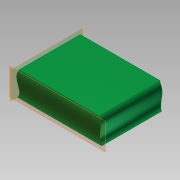
# Autodesk Inventor part: GP-WSM010 board
Saved by Autodesk Inventor 2011 (Build 150239000, 239)
## iProperties
Created: 2010-12-28
Part Number: GP-WSM010 board
Document SubType Name: Modeling
Designer: abbath
Density: 1 g/cm^3
Mass: 0.0283841 g
Surface Area: 0.648912 cm^2
Volume: 0.0283841 cm^3
Author: abbath
Autodesk Inventor part; units mm, degrees
ref_plane "YZ Plane" through (0, 0, 0) normal (1, 0, 0) x (0, 1, 0)
ref_plane "XZ Plane" through (0, 0, 0) normal (0, 1, 0) x (-1, 0, 0)
ref_plane "XY Plane" through (0, 0, 0) normal (0, 0, 1) x (1, 0, 0)
sketch "Эскиз1" plane through (0, 0, 0) normal (0, 0, 1) x (1, 0, 0)
  line L0 (-2.365, 1.705) -> (-2.365, -1.705) projected
  line L1 (-2.365, -1.705) -> (-1.665, -1.705) projected
  line L2 (2.365, 1.705) -> (1.665, 1.705) projected
  line L3 (2.365, -1.705) -> (2.365, 1.705) projected
  line L4 (-2.665, -2.005) -> (2.665, -2.005)
  line L5 (2.665, -2.005) -> (2.665, 2.005)
  line L6 (2.665, 2.005) -> (-2.665, 2.005)
  line L7 (-2.665, 2.005) -> (-2.665, -2.005)
  point P0 (0, 0)
  dimension "d0" = 0.3
  dimension "d1" = 0.3
  dimension "d2" = 0.3
  dimension "d3" = 0.3
  constraints: 8 end point, 2 parallel, 1 horizontal, 1 perpendicular
  measures "d0" distance between parallel lines of L0 L7
  measures "d1" distance between parallel lines of L4 L1
  measures "d2" distance between parallel lines of L6 L2
  measures "d3" distance between parallel lines of L5 L3
extrude "Выдавливание1" add sketch "Эскиз1" along normal blind 1.5
ref_plane "РабПлоскость1" through (-2.665, 2.005, 0) normal (-1, 0, 0) x (0, -1, 0)
ref_plane "РабПлоскость2" through (-2.665, -2.005, 0) normal (0, -1, 0) x (1, 0, 0)
sketch "Эскиз2" plane through (-2.665, -2.005, 0) normal (0, -1, 0) x (1, 0, 0)
  line L0 (5.33, 1.5) -> (0, 1.5) projected
  line L1 (0, 0) -> (0, 1.5) projected
  line L2 (0, 0) -> (5.33, 0) projected
  line L3 (5.33, 0) -> (5.33, 1.5) projected
  spline S0 degree 3 poles (5.2449, 0) (4.7317, 0.2339) (5.5909, 1.213) (5.0567, 1.5) knots 0 0 0 0 1 1 1 1
  spline S1 degree 3 poles (0.0711, 0) (0.2805, 0.1803) (-0.0864, 1.0499) (0.1661, 1.5) knots 0 0 0 0 1 1 1 1
  point P0 (2.665, 0)
  point P1 (5.0772, 0.3564)
  point P2 (5.2329, 1.0651)
  point P3 (0.1387, 0.2211)
  point P4 (0.0821, 0.8519)
  constraints: 4 point on line, 8 other
extrude "Выдавливание2" cut sketch "Эскиз2" against normal through all contours L3 L2 S0 L0 | S1 L2 L1 L0
sketch "Эскиз3" plane through (-2.665, 2.005, 0) normal (-1, 0, 0) x (0, -1, 0)
  line L0 (0, 0) -> (0, 1.5) projected
  line L1 (4.01, 0) -> (0, 0) projected
  line L2 (4.01, 1.5) -> (4.01, 0) projected
  line L3 (0, 1.5) -> (4.01, 1.5) projected
  spline S0 degree 3 poles (3.8642, 0) (3.6548, 0.359) (4.0728, 1.0978) (3.8351, 1.5) knots 0 0 0 0 1 1 1 1
  spline S1 degree 3 poles (0.1988, 0) (-0.208, 0.3173) (0.3844, 1.4102) (0.1, 1.5) knots 0 0 0 0 1 1 1 1
  point P0 (2.005, 0)
  point P1 (3.8109, 0.4111)
  point P2 (3.9029, 1.023)
  point P3 (0.0634, 0.5877)
  point P4 (0.1805, 1.327)
  constraints: 4 point on line, 8 other
extrude "Выдавливание3" cut sketch "Эскиз3" against normal through all contours L0 L3 S1 L1 | S0 L3 L2 L1
